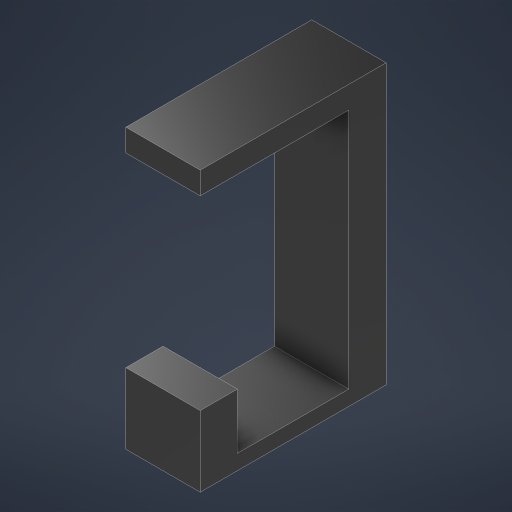
# Autodesk Inventor part: Hook
Saved by Autodesk Inventor 2023.6 (Build 276521000, 521)
## iProperties
Created: 2026-03-05
Part Number: Hook
Material: Generic
Document SubType Name: Modeling
Designer: user
Density: 1 g/cm^3
Appearance: Glossy - Black
Author: user
Autodesk Inventor part; units mm, degrees
ref_plane "YZ Plane" through (0, 0, 0) normal (1, 0, 0) x (0, 1, 0)
ref_plane "XZ Plane" through (0, 0, 0) normal (0, 1, 0) x (-1, 0, 0)
ref_plane "XY Plane" through (0, 0, 0) normal (0, 0, 1) x (1, 0, 0)
sketch "Sketch1" plane through (0, 0, 0) normal (1, 0, 0) x (0, 1, 0)
  line L0 (0, 0) -> (0, -6)
  line L1 (0, -6) -> (13, -6)
  line L2 (0, 0) -> (3, 0)
  line L3 (3, 0) -> (3, 2)
  line L4 (3, 2) -> (1.1991, 2)
  line L5 (1.1991, 2) -> (-0.8009, 2)
  line L6 (-0.8009, 2) -> (-0.8009, -8)
  line L7 (-0.8009, -8) -> (14.1991, -8)
  line L8 (0, -3) -> (14.1991, -3)
  line L9 (14.1991, -8) -> (14.1991, -3)
  line L10 (13, -6) -> (13, -3)
  line L11 (14.1991, -3) -> (14.1991, 2)
  line L12 (14.1991, 2) -> (13, 2)
  line L13 (13, 2) -> (13, -3)
  line L14 (14.1991, -3) -> (13.349, -3)
  dimension "d0" = 6
  dimension "d1" = 13
  dimension "d2" = 2
  dimension "d3" = 2
  dimension "d4" = 10
  dimension "d5" = 15
  dimension "d6" = 5
  constraints: 30 end point, 8 perpendicular, 4 horizontal, 3 point on line, 2 vertical, 1 midpoint
  measures "d0" distance of L0.start L0.end
  measures "d1" distance of L0.end L1.end
  measures "d2" distance of L2.end L3.end
  measures "d3" distance of L4.end L5.end
  measures "d4" distance of L5.end L6.end
  measures "d5" distance of L6.end L7.end
  measures "d6" distance of L8.end L11.end
extrude "Extrusion1" add sketch "Sketch1" along normal blind 4 contours L0 L1 L10 L8 L9 L7 L6 L5 L4 L3 L2 | L13 L12 L11 L8
body "Solid1"
